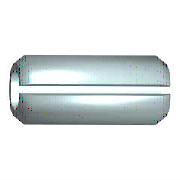
# Autodesk Inventor part: ISO 8752 - 3 x 6
Saved by Autodesk Inventor 2012 SP2 (Build 160219200, 219)
## iProperties
Created: 2011-02-07
Part Number: ISO 8752 - 3 x 6
Material: 不銹鋼，奧氏體
Description: 彈簧型直銷
Document SubType Name: Modeling
Standard: ISO 8752
Designer: ERIC
Standards Organization: DIN
Language: zh-TW
Size Designation: 3 x 6
Categories: <MemberInstance><Categories><Category DisplayName="結件" InternalName="e4da775c-781d-43d5-af7c-5136215cf5a6" Mnemonic="FSTN"><Category DisplayName="銷" InternalName="3b3d1810-ac9b-4ede-8c7f-cc6b956350b0" Mnemonic="PIN"><CategoryParameter DisplayName="標稱直徑" InternalName="6cc331d7-8ea1-4fca-9c9a-55ec966217e5" Mnemonic="nomdia"/><CategoryParameter DisplayName="標稱長度" InternalName="897bd938-6adf-4e3c-a2d4-0d7cae45eecd" Mnemonic="nomlen"/><Category DisplayName="圓柱" InternalName="f4e44bba-8648-4014-94fb-0d911bed22aa" Mnemonic="CYLPIN"><CategoryParameter DisplayName="實用長度" InternalName="4313d7a4-b766-4ddf-a49b-c6b4c6469386" Mnemonic="fnclen"/><CategoryParameter DisplayName="類型" InternalName="e2d46644-2f7a-4f6c-8641-d32369dac357" Mnemonic="type"/><CategoryParameter DisplayName="展開直徑" InternalName="10e07583-5af5-45d4-865e-34eee3987d42" Mnemonic="expanddia"/><CategoryParameter DisplayName="壁厚度" InternalName="ea9afbee-e724-4de7-9629-c276aafee907" Mnemonic="wllthick"/><CategoryParameter DisplayName="公差類別" InternalName="646c7720-a97e-458a-995e-628342705102" Mnemonic="tolerclss"/></Category></Category></Category><Category DisplayName="資料類型" InternalName="23b78d0f-2648-40c6-8793-ca6db495c9e8" Mnemonic="DATATYPE"><CategoryParameter DisplayName="顯示名稱" InternalName="05415f3d-3907-474b-a020-eb9d644f4cf3" Mnemonic="DISPLAYNAME"/><CategoryParameter DisplayName="內部名稱" InternalName="cf1d0246-76d9-4b4a-8305-fa0409afb5c1" Mnemonic="INTERNALNAME"/><CategoryParameter DisplayName="資料夾名稱" InternalName="3f06958e-8713-4116-9be7-ed6184ecc97b" Mnemonic="FOLDERNAME"/><CategoryParameter DisplayName="族群版本" InternalName="914462f6-6e19-4b14-ba84-155b9680b1d0" Mnemonic="FAMILYREVISION"/><CategoryParameter DisplayName="截取格式" InternalName="bc51e27b-3422-4e78-93ef-cec197ddf230" Mnemonic="CLIPFORMAT"/><CategoryParameter DisplayName="IsMetric" InternalName="e2385c5b-1ea4-4823-96a8-8de651266ec3" Mnemonic="ISMETRIC"/><CategoryParameter DisplayName="說明" InternalName="13903e3d-64b1-4950-80da-f627842ea37f" Mnemonic="DESCRIPTION"/><CategoryParameter DisplayName="標準組織" InternalName="8f5914e1-4693-403f-8ab5-d37768198c9d" Mnemonic="STDSORG"/><CategoryParameter DisplayName="標準" InternalName="0c0a119c-1e12-4c84-803f-101930972f5e" Mnemonic="STANDARD"/><CategoryParameter DisplayName="製造商" InternalName="cd6c7a72-a28a-4e50-99a9-2c7f4e13e5ad" Mnemonic="MANUFACTURER"/><CategoryParameter DisplayName="成員修訂" InternalName="a65d44b9-392f-4f4f-857b-e4b3d54996fe" Mnemonic="MEMBERREVISION"/><CategoryParameter DisplayName="標準版序" InternalName="91d5a463-65c2-4fde-b823-3b7fea5e8e17" Mnemonic="STANDARDREVISION"/><CategoryParameter DisplayName="版序指南" InternalName="45a75005-10b1-4dfc-8d6d-dfe629f0b93c" Mnemonic="REVISIONGUID"/><CategoryParameter DisplayName="稱號" InternalName="2675968c-4ce5-49e0-a4f5-552d29089031" Mnemonic="DESIGNATION"/><CategoryParameter DisplayName="檔案名稱" InternalName="8b46a4cc-9585-4fed-90c3-899f57e09a73" Mnemonic="FILENAME"/><CategoryParameter DisplayName="預設列" InternalName="2af9ec52-faaa-4026-b378-f9fa4afca842" Mnemonic="DEFAULTROW"/><Category DisplayName="零件" InternalName="c0e0b642-3bcb-4cc8-9e80-f96d35c4afa4" Mnemonic="PART"><CategoryParameter DisplayName="材料" InternalName="818a152a-d3c3-49ca-80ee-df7d91421b8e" Mnemonic="MATERIAL"/><CategoryParameter DisplayName="材料鍵" InternalName="5c9a8adb-dd2b-4535-b97f-0a94a95fe41f" Mnemonic="MATERIALKEY"/><CategoryParameter DisplayName="零件號碼" InternalName="016b6077-bfbe-49bd-92c9-d8d59c39c941" Mnemonic="PARTNUMBER"/><CategoryParameter DisplayName="庫存號碼" InternalName="4dba7c1c-e26c-444e-836c-b08b433409a8" Mnemonic="STOCKNUMBER"/></Category></Category><Category DisplayName="以前版本中參數映射" InternalName="cd87c42b-3e48-431e-b5c0-1cbeb14dfe77" Mnemonic="LEGACYMAP"><CategoryParameter DisplayName="目錄名稱" InternalName="d99d1e27-aa94-4de2-af4c-c348882a6f4f" Mnemonic="CATALOGNAME"/><CategoryParameter DisplayName="族群號碼" InternalName="e705e1f4-09cb-413e-91f9-551b4188271e" Mnemonic="FAMILYNUMBER"/><CategoryParameter DisplayName="成員 ID" InternalName="8e5e0294-fc51-4c8f-b3d7-003dc5ed94f6" Mnemonic="MEMBERID"/><CategoryParameter DisplayName="唯一 CC 成員 ID" InternalName="5193edd4-b2b0-4ab4-9d54-de900eee34e0" Mnemonic="CCCOOKIE"/><CategoryParameter DisplayName="唯一 DA 成員 ID" InternalName="0918ad47-427f-4fed-ae26-24c81c58f590" Mnemonic="DACOOKIE"/><CategoryParameter DisplayName="合併11 ID" InternalName="0ee8fb18-e2ed-4f39-96f6-1f4b5f50aa71" Mnemonic="MERGE11"/><CategoryParameter DisplayName="分割 ID" InternalName="72b5c83c-be7f-45c4-ae51-9160ea6deb26" Mnemonic="SPLIT"/></Category></Categories><FamilyTemplate Id="si0085_a"><FamilyTemplateParameters><FamilyTemplateParameter ObjectType="kUserParameterObject" ValueType="xs:double" Id="1" ObjectReferenceKey="NND1"/><FamilyTemplateParameter ObjectType="kUserParameterObject" ValueType="xs:double" Id="2" ObjectReferenceKey="PHH"/><FamilyTemplateParameter ObjectType="kUserParameterObject" ValueType="xs:double" Id="3" ObjectReferenceKey="SD"/><FamilyTemplateParameter ObjectType="kUserParameterObject" ValueType="xs:double" Id="4" ObjectReferenceKey="PHH1"/><FamilyTemplateParameter ObjectType="kUserParameterObject" ValueType="xs:double" Id="5" ObjectReferenceKey="FAWI"/><FamilyTemplateParameter ObjectType="kUserParameterObject" ValueType="xs:double" Id="6" ObjectReferenceKey="NND"/><FamilyTemplateParameter ObjectType="kUserParameterObject" ValueType="xs:double" Id="7" ObjectReferenceKey="NLG"/><FamilyTemplateParameter ObjectType="kPropertyObject" ValueType="xs:string" Id="100" ObjectReferenceKey="{32853F0F-3444-11d1-9E93-0060B03C1CA6}" SubObjectId="52"/><FamilyTemplateParameter ObjectType="kPropertyObject" ValueType="xs:string" Id="105" ObjectReferenceKey="{32853F0F-3444-11d1-9E93-0060B03C1CA6}" SubObjectId="5"/><FamilyTemplateParameter ObjectType="kPartComponentDefinitionObject" ValueType="xs:string" Id="110" SubObjectId="Material"/></FamilyTemplateParameters></FamilyTemplate><CategoryParameterMap><ParamToTemplateMap><ParamToTemplate CategoryParameter="//CategoryParameter[@InternalName='05415f3d-3907-474b-a020-eb9d644f4cf3']" ConstantValue="DIN EN ISO 8752"/><ParamToTemplate CategoryParameter="//CategoryParameter[@InternalName='cf1d0246-76d9-4b4a-8305-fa0409afb5c1']" ConstantValue="0ba0f8b9-414c-46cf-b9fe-67228a21c59e"/><ParamToTemplate CategoryParameter="//CategoryParameter[@InternalName='3f06958e-8713-4116-9be7-ed6184ecc97b']" ConstantValue="ISO 8752(2)"/><ParamToTemplate CategoryParameter="//CategoryParameter[@InternalName='914462f6-6e19-4b14-ba84-155b9680b1d0']" ConstantValue="10"/><ParamToTemplate CategoryParameter="//CategoryParameter[@InternalName='bc51e27b-3422-4e78-93ef-cec197ddf230']" ConstantValue="CF_INVENTOR.STDPARTS"/><ParamToTemplate CategoryParameter="//CategoryParameter[@InternalName='e2385c5b-1ea4-4823-96a8-8de651266ec3']" ConstantValue="true"/><ParamToTemplate CategoryParameter="//CategoryParameter[@InternalName='13903e3d-64b1-4950-80da-f627842ea37f']" ConstantValue="Spring-Type Straight Pin"/><ParamToTemplate CategoryParameter="//CategoryParameter[@InternalName='8f5914e1-4693-403f-8ab5-d37768198c9d']" ConstantValue="DIN"/><ParamToTemplate CategoryParameter="//CategoryParameter[@InternalName='0c0a119c-1e12-4c84-803f-101930972f5e']" ConstantValue="ISO 8752"/><ParamToTemplate CategoryParameter="//CategoryParameter[@InternalName='cd6c7a72-a28a-4e50-99a9-2c7f4e13e5ad']" TemplateParameter="104"/><ParamToTemplate CategoryParameter="//CategoryParameter[@InternalName='91d5a463-65c2-4fde-b823-3b7fea5e8e17']" TemplateParameter="103"/><ParamToTemplate CategoryParameter="//CategoryParameter[@InternalName='45a75005-10b1-4dfc-8d6d-dfe629f0b93c']" ConstantValue="7a7ad295-9682-47a3-adab-bb27b85750e6"/><ParamToTemplate CategoryParameter="//CategoryParameter[@InternalName='2af9ec52-faaa-4026-b378-f9fa4afca842']" ConstantValue="10"/><ParamToTemplate CategoryParameter="//CategoryParameter[@InternalName='d99d1e27-aa94-4de2-af4c-c348882a6f4f']" ConstantValue="DIN"/><ParamToTemplate CategoryParameter="//CategoryParameter[@InternalName='e705e1f4-09cb-413e-91f9-551b4188271e']" ConstantValue="213"/><ParamToTemplate CategoryParameter="//CategoryParameter[@InternalName='8b46a4cc-9585-4fed-90c3-899f57e09a73']" ConstantValue="ISO 8752 - 3 x 6  (2) DIN EN ISO"/><ParamToTemplate CategoryParameter="//CategoryParameter[@InternalName='a65d44b9-392f-4f4f-857b-e4b3d54996fe']" ConstantValue="b309a60a-7e1b-4bf3-9339-1a6be35082e8"/><ParamToTemplate CategoryParameter="//CategoryParameter[@InternalName='e2d46644-2f7a-4f6c-8641-d32369dac357']" ConstantValue=""/><ParamToTemplate CategoryParameter="//CategoryParameter[@InternalName='4313d7a4-b766-4ddf-a49b-c6b4c6469386']" ConstantValue="3.76077"/><ParamToTemplate CategoryParameter="//CategoryParameter[@InternalName='8e5e0294-fc51-4c8f-b3d7-003dc5ed94f6']" ConstantValue="530"/><ParamToTemplate CategoryParameter="//CategoryParameter[@InternalName='2675968c-4ce5-49e0-a4f5-552d29089031']" TemplateParameter="100"/><ParamToTemplate CategoryParameter="//CategoryParameter[@InternalName='818a152a-d3c3-49ca-80ee-df7d91421b8e']" TemplateParameter="110"/><ParamToTemplate CategoryParameter="//CategoryParameter[@InternalName='897bd938-6adf-4e3c-a2d4-0d7cae45eecd']" TemplateParameter="7"/><ParamToTemplate CategoryParameter="//CategoryParameter[@InternalName='6cc331d7-8ea1-4fca-9c9a-55ec966217e5']" TemplateParameter="6"/><ParamToTemplate CategoryParameter="//CategoryParameter[@InternalName='016b6077-bfbe-49bd-92c9-d8d59c39c941']" TemplateParameter="105"/></ParamToTemplateMap></CategoryParameterMap></MemberInstance>
Density: 8.03 g/cm^3
IsCustomPart: 1
Author: ERIC
Autodesk Inventor part; units mm, degrees
ref_plane "YZ Plane" through (0, 0, 0) normal (1, 0, 0) x (0, 1, 0)
ref_plane "XZ Plane" through (0, 0, 0) normal (0, 1, 0) x (-1, 0, 0)
sketch "草圖1" plane through (0, 0, 0) normal (0, 0, 1) x (1, 0, 0)
  line L0 (0, 1.15) -> (0, 1.616)
  line L1 (0, 1.616) -> (0.5, 1.75)
  line L2 (0.5, 1.75) -> (5.5, 1.75)
  line L3 (5.5, 1.75) -> (6, 1.616)
  line L4 (6, 1.616) -> (6, 1.15)
  line L5 (6, 0) -> (0, 0)
  line L6 (0, 1.15) -> (6, 1.15)
  line L7 (0, 1.15) -> (0, 0) construction
  line L8 (6, 1.15) -> (6, 0) construction
  line L9 (0, 1.68) -> (0, -0.28) projected
  line L10 (-2, 0) -> (12, 0) projected
  dimension "d0" = 6
  dimension "d1" = 3.5
  dimension "d2" = 2.3
  dimension "d3" = 15
  dimension "d4" = 15
  dimension "d7" = 0.134
  dimension "d8" = 0.134
  constraints: 18 end point, 3 parallel, 3 perpendicular, 1 coincident, 1 point on line, 1 vertical
  measures "d0" distance between parallel lines of L4 L0
  measures "d1" diameter of L2 L5
  measures "d2" diameter of L6 L5
  measures "d3" angle of L2 L1
  measures "d4" angle of L3 L2
  measures "d7" vertical distance of L1.end L0.end
  measures "d8" vertical distance of L2.end L3.end
revolve "本體" add sketch "草圖1" angle 360 about axis through (6, 0, 0) along (-1, 0, 0)
ref_plane "Work Plane1" through (3, 0, 0) normal (1, 0, 0) x (0, 1, 0)
sketch "草圖2" plane through (3, 0, 0) normal (1, 0, 0) x (0, 1, 0)
  arc A0 (0.2193, 1.7362) -> (-0.2193, 1.7362) centre (0, 0) ccw
  arc A1 (0.1441, 1.1409) -> (-0.1441, 1.1409) centre (0, 0) ccw
  line L0 (-0.1441, 1.1409) -> (-0.2193, 1.7362)
  line L1 (0.1441, 1.1409) -> (0.2193, 1.7362)
  line L2 (0, 1.68) -> (0, -0.28) projected
  line L3 (-0.2457, 0) -> (0.2457, 0) projected
  dimension "d11" = 1.75
  dimension "d12" = 1.15
  dimension "d14" = 0.6
  dimension "d15" = 7.2
  constraints: 4 end point, 4 point on circle, 2 centre point, 2 coincident, 2 horizontal alignment, 1 other
  measures "d11" radius of A0
  measures "d12" radius of A1
  measures "d14" distance of L0.start L0.end
  measures "d15" angle of L2 L0
extrude "切割" cut sketch "草圖2" against normal mid plane 6
equation "\"d11\" = 0.5 * NND1"
equation "\"d12\" = -SD + 0.5 * NND1"
equation "\"d14\" = SD"
equation "\"d5\" = NLG"
equation "\"d0\" = NLG"
equation "\"d1\" = NND1"
equation "\"d2\" = NND1 - 2 * SD"
equation "\"d3\" = FAWI"
equation "\"d4\" = FAWI"
equation "\"NND\" = 3"
equation "\"NLG\" = 6"
equation "\"SD\" = 0.6"
equation "\"PHH\" = 0.5"
equation "\"PHH1\" = PHH"
equation "\"FAWI\" = 15deg"
equation "\"d9\" = 0.5 * NLG"
equation "\"NND1\" = 3.5"
body "Solid1"
